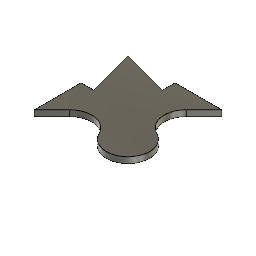
ringing_vfa_01 (Autodesk Fusion 360 design; units mm, degrees)
Autodesk Fusion 360 part; units mm, degrees
sketch "Sketch1" plane through (0, 0, 0) normal (0, 0, 1) x (1, 0, 0)
  line L0 (0, 0) -> (0, 185) construction
  line L1 (0, 185) -> (-185, 185)
  line L2 (-185, 185) -> (-185, 0)
  line L3 (-185, 0) -> (0, 0) construction
  line L4 (-185, 0) -> (-149.6447, 35.3553)
  arc A0 (-81.0777, 23.933) -> (-149.6447, 35.3553) centre (-119.4412, 5.1519) ccw
  arc A1 (-81.0777, 23.933) -> (-23.933, 81.0777) centre (-42.7141, 42.7141) ccw
  arc A2 (-35.3553, 149.6447) -> (-23.933, 81.0777) centre (-5.1519, 119.4412) ccw
  line L5 (-35.3553, 149.6447) -> (0, 185)
  line L6 (0, 0) -> (-185, 185) construction
  line L7 (-185, 185) -> (-92.5, 160.2147)
  line L8 (-92.5, 160.2147) -> (-92.5, 185)
  line L9 (-185, 185) -> (-160.2147, 92.5)
  line L10 (-160.2147, 92.5) -> (-185, 92.5)
  dimension "d2" = 185
  dimension "d3" = 45
  dimension "d4" = 45
  dimension "d10" = 60
  dimension "d21" = 50
  constraint coincident L0.start L3.end
  constraint tangent L4 A0
  constraint tangent A2 L5
  constraint coincident A1.centre L6
  constraint equal L1 L2
  constraint perpendicular L1 L2
  constraint perpendicular L2 L3
  constraint perpendicular L0 L3
  constraint horizontal L3
  constraint coincident L1 L8.end
  constraint perpendicular L1 L8
  constraint coincident L2 L10.end
  constraint perpendicular L2 L10
  constraint symmetric L6 L7 L9
  constraint midpoint L1 L8.end
  constraint midpoint L2 L10.end
  constraint tangent L3 A1
  constraint equal A0 A1
  constraint coincident A0.start A1.start
  constraint coincident A1.end A2.end
  constraint tangent A0 A1
  constraint tangent A1 A2
  constraint equal A0 A2
  measures "d2" distance of L0.start L2.end
  measures "d3" angle of L3 L4
  measures "d4" angle of L0 L5
  measures "d10" angle of L7 L9
  measures "d21" distance of L2.end L4.end
extrude "Extrude1" add sketch "Sketch1" along normal blind 12 contours L1 L2 L4 A0 A1 A2 L5 L7 L8 L9 L10
